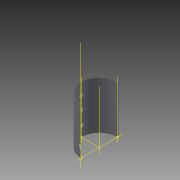
# Autodesk Inventor part: Upper Front Half 2014 Replacement
Saved by Autodesk Inventor 2015 (Build 190159000, 159)
## iProperties
Created: 2014-07-11
Part Number: Upper Front Half 2014 Replacement
Material: Generic
Document SubType Name: Modeling
Designer: I Rabey
Density: 1 g/cm^3
Appearance: Default
Author: I Rabey
Autodesk Inventor part; units mm, degrees
sketch "Sketch1" plane through (0, 0, 0) normal (0, 1, 0) x (-1, 0, 0)
  line L0 (0, 0) -> (0, 306) construction
  line L1 (0, 0) -> (0, -306) construction
  arc A0 (0, -308) -> (0, 308) centre (0, 0) ccw
  arc A1 (0, -307) -> (0, 307) centre (0, 0) ccw
  line L2 (0, 0) -> (0, -307) construction
  line L3 (0, 0) -> (0, 307) construction
  line L4 (0, -308) -> (0, -307)
  line L5 (0, 307) -> (0, 308)
  dimension "d1" = 180
  dimension "d2" = 308
  dimension "d124" = 307
  dimension "d125" = 180
  constraints: 12 end point, 4 point on circle, 3 coincident, 2 centre point, 2 vertical, 1 point on line
  measures "d1" angle of L0 L1
  measures "d2" radius of A0
  measures "d124" radius of A1
  measures "d125" angle of L2 L3
extrude "Extrusion1" add sketch "Sketch1" along normal blind 810.25
sketch "Sketch2" plane through (0, 0, 0) normal (0, 1, 0) x (-1, 0, 0)
  line L0 (0, -307) -> (1, -307)
  line L1 (1, -307) -> (1, -323)
  line L2 (1, -323) -> (0, -323)
  line L3 (0, -323) -> (0, -307)
  line L4 (0, 307.0245) -> (1, 307.0245)
  line L5 (1, 307.0245) -> (1, 323.0245)
  line L6 (1, 323.0245) -> (0, 323.0245)
  line L7 (0, 323.0245) -> (0, 307.0245)
  point P0 (0, 0)
  point P1 (0, 308)
  point P2 (0, -308)
  dimension "d152" = 1
  dimension "d153" = 16
  dimension "d154" = 1
  dimension "d155" = 16
  constraints: 16 end point, 4 parallel, 2 horizontal, 2 perpendicular
  measures "d152" distance of L1.end L2.end
  measures "d153" distance of L0.end L1.end
  measures "d154" distance of L6.end L5.end
  measures "d155" distance of L5.end L4.end
extrude "Extrusion2" add sketch "Sketch2" along normal blind 810.25
ref_plane "Work Plane7" through (-308, 0, 0) normal (-1, 0, 0) x (0, -1, 0)
ref_plane "Work Plane8" through (-1, 0, 307.9984) normal (-0.0032468, 0, 0.9999947) x (0.9999947, 0, 0.0032468)
ref_plane "Work Plane9" through (-1, 0, -307.9984) normal (-0.0032468, 0, -0.9999947) x (-0.9999947, 0, 0.0032468)
sketch "Sketch17" plane through (-308, 0, 0) normal (-1, 0, 0) x (0, -1, 0)
  circle A0 centre (-395.75, 0) radius 38.5
  line L0 (0, -307.9984) -> (0, 307.9984) projected
  circle A1 centre (-610.75, 0) radius 38.5
  circle A2 centre (-167.25, 0) radius 38.5
  point P0 (0, 0)
  dimension "d110" = 77
  dimension "d111" = 395.75
  dimension "d126" = 77
  dimension "d130" = 77
  dimension "d134" = 610.75
  dimension "d156" = 167.25
  constraints: 3 centre point
  measures "d110" diameter of A0
  measures "d111" distance from line of L0 A0.centre
  measures "d126" diameter of A1
  measures "d130" diameter of A2
  measures "d134" distance from line of L0 A1.centre
  measures "d156" distance from line of L0 A2.centre
extrude "Extrusion9" cut sketch "Sketch17" along normal blind 167.25 and the other way blind 20
sketch "Sketch20" plane through (-1, 0, 307.9984) normal (-0.0032468, 0, 0.9999947) x (0.9999947, 0, 0.0032468)
  line L0 (0, 0) -> (0, 810.25) projected
  circle A0 centre (0, 167.25) radius 38.5
  line L1 (0, 0) -> (-308, 0) projected
  point P0 (-2, 0)
  dimension "d157" = 77
  dimension "d158" = 167.25
  constraints: 1 centre point, 1 point on line
  measures "d157" diameter of A0
  measures "d158" distance from line of L1 A0.centre
extrude "Extrusion12" cut sketch "Sketch20" along normal blind 25 and the other way blind 25
equation "\"d136\" = d156"
body "Solid1"
